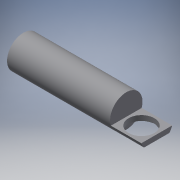
# Autodesk Inventor part: Ring Connector model 3
Saved by Autodesk Inventor 2017 (Build 210142000, 142)
## iProperties
Created: 2017-03-02
Part Number: Ring Connector model 3
Material: Generic
Document SubType Name: Modeling
Designer: coffmant
Density: 1 g/cm^3
Appearance: Default
Quantity: 1
Author: coffmant
Autodesk Inventor part; units mm, degrees
ref_plane "YZ Plane" through (0, 0, 0) normal (1, 0, 0) x (0, 1, 0)
ref_plane "XZ Plane" through (0, 0, 0) normal (0, 1, 0) x (-1, 0, 0)
ref_plane "XY Plane" through (0, 0, 0) normal (0, 0, 1) x (1, 0, 0)
sketch "Sketch1" plane through (0, 0, 0) normal (1, 0, 0) x (0, 1, 0)
  circle A0 centre (0, 0) radius 8.001
  dimension "d0" = 16.002
  constraints: 1 centre point, 1 coincident
  measures "d0" diameter of A0
extrude "Extrusion1" add sketch "Sketch1" along normal blind 50.8
sketch "Sketch2" plane through (50.8, 0, 0) normal (1, 0, 0) x (0, 0, -1)
  line L0 (-6.2432, -5.0038) -> (6.2432, -5.0038)
  line L1 (-7.5991, -2.5038) -> (7.5991, -2.5038)
  arc A0 (6.2432, -5.0038) -> (7.5991, -2.5038) centre (0, 0) ccw
  arc A1 (-7.5991, -2.5038) -> (-6.2432, -5.0038) centre (0, 0) ccw
  circle A2 centre (0, 0) radius 8.001 projected
  point P0 (7.0332, -3.8145)
  point P1 (-7.0332, -3.8145)
  dimension "d3" = 5.0038
  dimension "d4" = 2.5
  constraints: 12 point on circle, 4 end point, 2 centre point, 1 horizontal, 1 parallel
  measures "d3" distance from line of point (0, 0) L0
  measures "d4" distance between parallel lines of L0 L1
extrude "Extrusion2" add sketch "Sketch2" along normal blind 15.0114 contours A1 L1 A0 L0
sketch "Sketch3" plane through (50.8, -2.5038, 7.5991) normal (0, 1, 0) x (1, 0, 0)
  circle A0 centre (7.5057, 7.5991) radius 6.35
  line L0 (0, 15.1983) -> (15.0114, 15.1983) projected
  line L1 (0, 0) -> (15.0114, 0) projected
  point P0 (-50.8, 7.5991)
  point P1 (7.5057, 15.1983)
  dimension "d8" = 12.7
  dimension "d9" = 7.5991
  dimension "d10" = 15.1983
  constraints: 1 centre point, 1 midpoint, 1 vertical alignment
  measures "d8" diameter of A0
  measures "d9" distance from line of L0 A0.centre
  measures "d10" distance between parallel lines of L1 L0
extrude "Extrusion3" cut sketch "Sketch3" against normal blind 15.0114
equation "\"d9\" = 0.5 * d10"
body "Solid1"
